Autodesk Fusion 360 part; units mm, degrees
(part 2 of 2)
sketch "Livingroom_Sketche" plane through (0, 0, 0) normal (0, 0, 1) x (-1, 0, 0)
  line L0 (-255, -10) -> (-255, -140)
  line L1 (-255, -140) -> (-110, -140)
  line L2 (-110, -140) -> (-110, -130)
  line L3 (-110, -130) -> (-100, -130)
  line L4 (-100, -130) -> (-100, -170)
  line L5 (-100, -170) -> (-110, -170)
  line L6 (-110, -170) -> (-110, -160)
  line L7 (-110, -160) -> (-340, -160)
  line L8 (-340, -160) -> (-340, -340)
  line L9 (-340, -340) -> (-110, -340)
  line L10 (-110, -340) -> (-110, -250)
  line L11 (-110, -250) -> (-100, -250)
  line L12 (-100, -250) -> (-100, -280)
  line L13 (-100, -280) -> (0, -280)
  line L14 (0, -280) -> (0, -100)
  line L15 (0, -100) -> (10, -100)
  line L16 (10, -100) -> (10, -340)
  line L17 (10, -340) -> (340, -340)
  line L18 (340, -340) -> (340, -10)
  line L19 (340, -10) -> (10, -10)
  line L20 (10, -10) -> (10, -20)
  line L21 (10, -20) -> (0, -20)
  line L22 (0, -20) -> (0, 0)
  line L23 (0, 0) -> (350, 0)
  line L24 (350, 0) -> (350, 20)
  line L25 (350, 20) -> (365, 20)
  line L26 (365, 20) -> (365, 0)
  line L27 (365, 0) -> (420, 0)
  line L28 (420, 0) -> (480, 0)
  line L29 (480, 0) -> (480, 360)
  line L30 (480, 360) -> (365, 360)
  line L31 (365, 360) -> (365, 330)
  line L32 (365, 330) -> (350, 330)
  line L33 (350, 330) -> (350, 350)
  line L34 (350, 350) -> (13, 350)
  line L35 (13, 350) -> (13, 360)
  line L36 (13, 360) -> (-85, 360)
  line L37 (-85, 360) -> (-85, 350)
  line L38 (-85, 350) -> (-100, 350)
  line L39 (-100, 350) -> (-100, -50)
  line L40 (-100, -50) -> (-110, -50)
  line L41 (-110, -50) -> (-110, -10)
  line L42 (-110, -10) -> (-255, -10)
  line L43 (350, 0) -> (325, 0)
  line L44 (325, 0) -> (325, 20)
  line L45 (325, 20) -> (350, 20)
  line L46 (350, 20) -> (350, 0)
  line L47 (325, 20) -> (45, 20)
  line L48 (45, 20) -> (45, 85)
  line L49 (45, 85) -> (325, 85)
  line L50 (325, 85) -> (325, 20)
  line L51 (325, 85) -> (260, 85)
  line L52 (260, 85) -> (260, 195)
  line L53 (260, 195) -> (325, 195)
  line L54 (325, 195) -> (325, 85)
  line L55 (13, 350) -> (45, 350)
  line L56 (45, 350) -> (45, 275)
  line L57 (45, 275) -> (13, 275)
  line L58 (13, 275) -> (13, 350)
  line L59 (13, 350) -> (350, 350)
  line L60 (350, 350) -> (350, 330)
  line L61 (350, 330) -> (13, 330)
  line L62 (13, 330) -> (13, 350)
  line L63 (320, 85) -> (320, 25)
  line L64 (320, 25) -> (50, 25)
  line L65 (50, 25) -> (50, 85)
  dimension "d260" = 5
  constraint horizontal L43
  constraint vertical L44
  constraint horizontal L45
  constraint vertical L46
  constraint coincident L23.end L24.start
  constraint horizontal L47
  constraint vertical L48
  constraint horizontal L49
  constraint vertical L50
  constraint horizontal L51
  constraint vertical L52
  constraint horizontal L53
  constraint vertical L54
  constraint horizontal L55
  constraint vertical L56
  constraint horizontal L57
  constraint vertical L58
  constraint coincident L34.end L35.start
  constraint horizontal L59
  constraint vertical L60
  constraint horizontal L61
  constraint vertical L62
  constraint coincident L32.end L33.start
extrude "Extrude52" add sketch "Livingroom_Sketche" along normal blind 40 separate body contours L34 L55 L56 L58 L59 L61 L62 | L56 L57 L58 L61 makes body 20
extrude "Extrude53" add sketch "Livingroom_Sketche" along normal blind 320 contours L34 L55 L56 L58 L59 L61 L62 | L33 L34 L56 L59 L60 L61 bodies 20
sketch "Livingroom_TV1" plane through (0, -330, 0) normal (0, 1, 0) x (-1, 0, 0)
  line L0 (13, 40) -> (45, 40)
  line L1 (45, 40) -> (45, 0)
  line L2 (45, 0) -> (350, 0)
  line L3 (350, 0) -> (350, 320)
  line L4 (350, 320) -> (13, 320)
  line L5 (13, 320) -> (13, 40)
  line L6 (261, 152.5) -> (94, 152.5)
  line L7 (94, 152.5) -> (94, 57.5)
  line L8 (94, 57.5) -> (261, 57.5)
  line L9 (261, 57.5) -> (261, 152.5)
  line L10 (276, 167.5) -> (79, 167.5)
  line L11 (79, 167.5) -> (79, 42.5)
  line L12 (79, 42.5) -> (276, 42.5)
  line L13 (276, 42.5) -> (276, 167.5)
  line L14 (151.3931, 85) -> (215.3715, 85) construction
  line L15 (215.3715, 85) -> (215.3715, 117.3644) construction
  line L16 (215.3715, 117.3644) -> (151.3931, 117.3644) construction
  line L17 (151.3931, 117.3644) -> (151.3931, 85) construction
  point P0 (177.5, 105)
  dimension "d252" = 167
  dimension "d253" = 95
  dimension "d254" = 15
  dimension "d257" = 30
  text T0 "TV" font "Arial" height 30 align left top in box 63.9784 x 32.3644 at (151.3931, 85) x (1, 0) y (0, 1) spacing 1 kerned
  constraint horizontal L6
  constraint perpendicular L6 L7
  constraint parallel L6 L8
  constraint parallel L7 L9
  measures "d252" distance of L7.end L8.end
  measures "d253" distance of L6.end L7.end
extrude "Extrude54" cut sketch "Livingroom_TV1" along normal blind 19.8 contours L10 L11 L12 L13 bodies 20
sketch "Livingroom_TV2" plane through (0, -330, 0) normal (0, 1, 0) x (-1, 0, 0)
extrude "Extrude55" cut sketch "Livingroom_TV1" along normal blind 2 text T0 bodies 20
extrude "Extrude56" add sketch "Livingroom_Sketche" along normal blind 48 separate body contours L49 L51 L52 L53 L54 | L49 L51 L63 L64 L65 makes body 21
extrude "Extrude57" add sketch "Livingroom_Sketche" along normal blind 108 contours L47 L48 L49 L50 L51 L63 L64 L65 bodies 21
fillet "Fillet3" radius 36 2 edges at (-322.5, -85, 108) (-47.5, -85, 108) on bodies 21
extrude "Extrude58" cut sketch "Livingroom_TV1" against normal blind 19.8 contours L10 L11 L12 L13 bodies 20
extrude "Extrude59" cut sketch "Livingroom_TV1" against normal blind 2 text T0 bodies 20
draft "Draft1" [suppressed]
sketch "Sketch29" plane through (0, -10, 0) normal (0, -1, 0) x (1, 0, 0)
  line L0 (320, 0) -> (320, 320)
  line L1 (320, 320) -> (110, 320)
  line L2 (110, 320) -> (110, 310)
  line L3 (110, 310) -> (100, 310)
  line L4 (100, 310) -> (100, 5)
  line L5 (100, 5) -> (110, 5)
  line L6 (110, 5) -> (110, 0)
  line L7 (110, 0) -> (320, 0)
  line L8 (160, 75) -> (160, 105)
  line L9 (160, 105) -> (285, 105)
  constraint vertical L8
  constraint perpendicular L8 L9
named bodies: "Frame", "Floor", "Wardrobe", "Bedside_Table", "Bed", "Kitchen_Door1", "Kitchen_Door2", "Fridge", "Kitchen_Stove_Washbasin", "Kitchen_Cupboard", "Kitchen_Microwave", "Kitchen_Baker", "Kitchen_Water_Boil", "Kitchen_Dishwasher", "Kitchen_Clothewasher", "Holder", "Kitchen_Range_hood", "Kitchen_Range_Hood_Cupboard", "Studyroom_table", "Livingroom_TV", "Livingroom_Sofa"
